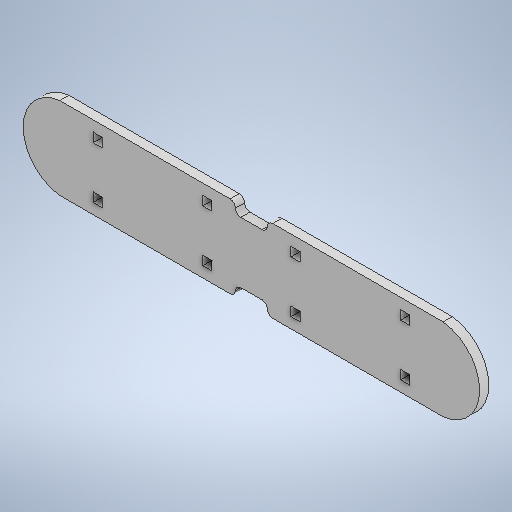
# Autodesk Inventor part: ASA_SUPERIOR
Saved by Autodesk Inventor 2025.1 (Build 291241000, 241)
## iProperties
Created: 2024-10-18
Part Number: ASA_SUPERIOR
Material: Genérico
Document SubType Name: Modeling
Designer: ambrosildo
Density: 1 g/cm^3
Appearance: Padrão
Author: ambrosildo
Autodesk Inventor part; units mm, degrees
ref_plane "YZ Plane" through (0, 0, 0) normal (1, 0, 0) x (0, 1, 0)
ref_plane "XZ Plane" through (0, 0, 0) normal (0, 1, 0) x (-1, 0, 0)
ref_plane "XY Plane" through (0, 0, 0) normal (0, 0, 1) x (1, 0, 0)
sketch "Esboço1" plane through (0, 0, 0) normal (0, 0, 1) x (1, 0, 0)
  arc A0 (-63, 13.5) -> (-75, 0) centre (-61.4063, 0) ccw
  line L0 (0, 10) -> (-3.5, 10)
  arc A1 (-5.25, 11.75) -> (-7, 13.5) centre (-7, 11.75) ccw
  arc A2 (-5.25, 11.75) -> (-3.5, 10) centre (-3.5, 11.75) ccw
  line L1 (-7, 13.5) -> (-63, 13.5)
  line L2 (-49, 10) -> (-52, 10)
  line L3 (-52, 10) -> (-52, 7)
  line L4 (-52, 7) -> (-49, 7)
  line L5 (-49, 7) -> (-49, 10)
  line L6 (-13, 10) -> (-16, 10)
  line L7 (-16, 10) -> (-16, 7)
  line L8 (-16, 7) -> (-13, 7)
  line L9 (-13, 7) -> (-13, 10)
  line L10 (0, 10) -> (3.5, 10)
  arc A3 (3.5, 10) -> (5.25, 11.75) centre (3.5, 11.75) ccw
  arc A4 (7, 13.5) -> (5.25, 11.75) centre (7, 11.75) ccw
  line L11 (7, 13.5) -> (63, 13.5)
  arc A5 (75, 0) -> (63, 13.5) centre (61.4063, 0) ccw
  line L12 (49, 10) -> (52, 10)
  line L13 (52, 10) -> (52, 7)
  line L14 (52, 7) -> (49, 7)
  line L15 (49, 7) -> (49, 10)
  line L16 (13, 10) -> (16, 10)
  line L17 (16, 10) -> (16, 7)
  line L18 (16, 7) -> (13, 7)
  line L19 (13, 7) -> (13, 10)
  line L20 (0, -10) -> (-3.5, -10)
  arc A6 (-3.5, -10) -> (-5.25, -11.75) centre (-3.5, -11.75) ccw
  arc A7 (-7, -13.5) -> (-5.25, -11.75) centre (-7, -11.75) ccw
  line L21 (-7, -13.5) -> (-63, -13.5)
  arc A8 (-75, 0) -> (-63, -13.5) centre (-61.4063, 0) ccw
  line L22 (-49, -10) -> (-52, -10)
  line L23 (-52, -10) -> (-52, -7)
  line L24 (-52, -7) -> (-49, -7)
  line L25 (-49, -7) -> (-49, -10)
  line L26 (-13, -10) -> (-16, -10)
  line L27 (-16, -10) -> (-16, -7)
  line L28 (-16, -7) -> (-13, -7)
  line L29 (-13, -7) -> (-13, -10)
  arc A9 (63, -13.5) -> (75, 0) centre (61.4063, 0) ccw
  line L30 (52, -10) -> (52, -7)
  line L31 (49, -10) -> (52, -10)
  line L32 (52, -7) -> (49, -7)
  line L33 (49, -7) -> (49, -10)
  line L34 (7, -13.5) -> (63, -13.5)
  line L35 (16, -10) -> (16, -7)
  line L36 (16, -7) -> (13, -7)
  line L37 (13, -10) -> (16, -10)
  line L38 (13, -7) -> (13, -10)
  arc A10 (5.25, -11.75) -> (7, -13.5) centre (7, -11.75) ccw
  arc A11 (5.25, -11.75) -> (3.5, -10) centre (3.5, -11.75) ccw
  line L39 (0, -10) -> (3.5, -10)
  point P0 (0, 0)
  dimension "d6" = 3.5
  constraints: 80 end point, 24 point on circle, 12 centre point, 4 parallel, 3 horizontal, 2 perpendicular
  measures "d6" distance between parallel lines of L11 L12
extrude "Extrusão1" add sketch "Esboço1" along normal blind 3
